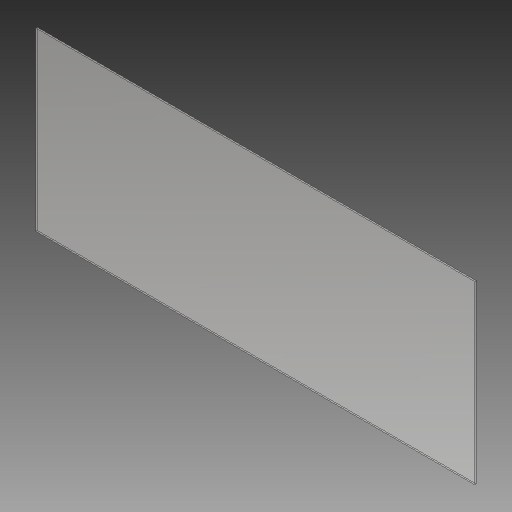
# Autodesk Inventor part: Plexi Glass
Saved by Autodesk Inventor 2019 (Build 230136000, 136)
## iProperties
Created: 2019-02-14
Part Number: Plexi Glass
Material: Generic
Document SubType Name: Modeling
Designer: josh
Density: 1 g/cm^3
Appearance: Clear
Mass: 573.822 g
Surface Area: 4571.7 cm^2
Volume: 573.822 cm^3
Author: josh
Autodesk Inventor part; units mm, degrees
ref_plane "YZ Plane" through (0, 0, 0) normal (1, 0, 0) x (0, 1, 0)
ref_plane "XZ Plane" through (0, 0, 0) normal (0, 1, 0) x (-1, 0, 0)
ref_plane "XY Plane" through (0, 0, 0) normal (0, 0, 1) x (1, 0, 0)
sketch "Sketch1" plane through (0, 0, 0) normal (0, 0, 1) x (1, 0, 0)
  line L0 (0, 0) -> (750.57, 0)
  line L1 (750.57, 0) -> (750.57, 300.99)
  line L2 (750.57, 300.99) -> (0, 300.99)
  line L3 (0, 300.99) -> (0, 0)
  dimension "d0" = 750.57
  dimension "d1" = 300.99
  constraints: 8 end point, 2 parallel, 1 horizontal, 1 perpendicular
  measures "d0" distance of L2.end L1.end
  measures "d1" distance of L0.end L1.end
extrude "Extrusion1" add sketch "Sketch1" along normal blind 2.54
body "Solid1"
